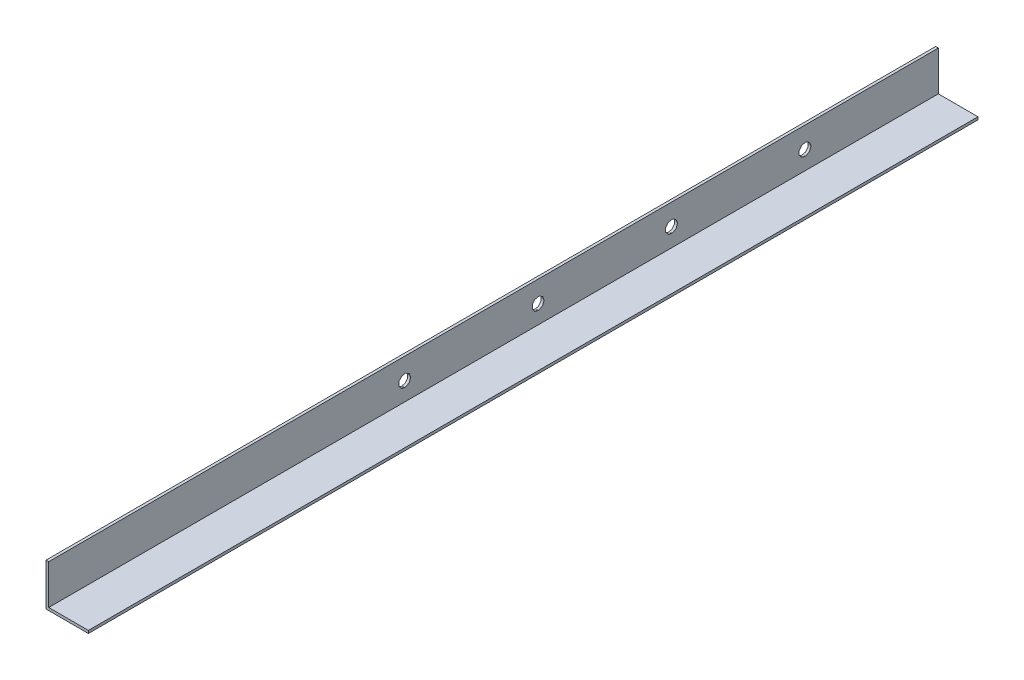
# Autodesk Inventor part: angle al 1.5x1.5 (48)
Saved by Autodesk Inventor 2015 (Build 190159000, 159)
## iProperties
Created: 2015-01-11
Part Number: angle al 1.5x1.5 (48)
Material: Generic
Document SubType Name: Modeling
Designer: chapale16
Density: 1 g/cm^3
Appearance: Default
Author: chapale16
Autodesk Inventor part; units mm, degrees
ref_plane "YZ Plane" through (0, 0, 0) normal (1, 0, 0) x (0, 1, 0)
ref_plane "XZ Plane" through (0, 0, 0) normal (0, 1, 0) x (-1, 0, 0)
ref_plane "XY Plane" through (0, 0, 0) normal (0, 0, 1) x (1, 0, 0)
sketch "Sketch1" plane through (0, 0, 0) normal (0, 0, 1) x (1, 0, 0)
  line L0 (0, 0) -> (0, -50.8)
  line L1 (0, -50.8) -> (50.8, -50.8)
  line L2 (3.2258, 0) -> (3.2258, -47.5742)
  line L3 (3.2258, -47.5742) -> (50.8, -47.5742)
  line L4 (0, 0) -> (3.2258, 0)
  line L5 (50.8, -47.5742) -> (50.8, -50.8)
  dimension "d0" = 50.8
  dimension "d1" = 50.8
  dimension "d2" = 3.2258
  constraints: 12 end point, 3 perpendicular, 1 horizontal, 1 vertical, 1 other
  measures "d0" distance of L0.start L0.end
  measures "d1" distance of L0.end L1.end
  measures "d2" distance between parallel lines of L0 L2
extrude "Extrusion1" add sketch "Sketch1" along normal blind 1066.8
sketch "Sketch2" plane through (0, -50.8, 0) normal (-1, 0, 0) x (0, 0, 1)
  line L0 (1066.8, 50.8) -> (1066.8, 0) projected
  line L1 (0, 50.8) -> (0, 0) projected
  point P0 (160.02, 25.4)
  point P1 (320.04, 25.4)
  point P2 (480.06, 25.4)
  point P3 (640.08, 25.4)
  dimension "d5" = 1066.8
  measures "d5" distance between parallel lines of L0 L1
hole "Hole1" at (0, -25.4, 480.06) at (0, -25.4, 640.08) at (0, -25.4, 320.04) at (0, -25.4, 160.02) direction (1, 0, 0) diameter 14.605 end through all
sketch "Sketch3" plane through (0, -50.8, 0) normal (-1, 0, 0) x (0, 0, 1)
  point P0 (0, 50.8)
  point P1 (797.56, 25.4)
  point P2 (957.58, 25.4)
body "Solid1"
